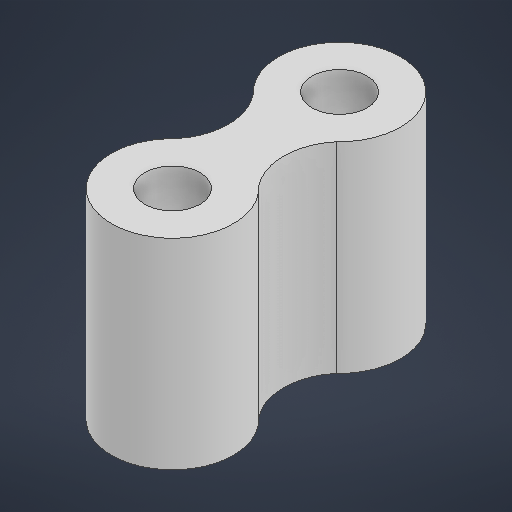
# Autodesk Inventor part: extBoardSpacer
Saved by Autodesk Inventor 2026 (Build 300175000, 175)
## iProperties
Created: 2025-05-16
Part Number: extBoardSpacer
Material: Generic
Document SubType Name: Modeling
Designer: Elizabeth
Density: 1 g/cm^3
Appearance: Default
Author: Elizabeth
Autodesk Inventor part; units mm, degrees
ref_plane "YZ Plane" through (0, 0, 0) normal (1, 0, 0) x (0, 1, 0)
ref_plane "XZ Plane" through (0, 0, 0) normal (0, 1, 0) x (-1, 0, 0)
ref_plane "XY Plane" through (0, 0, 0) normal (0, 0, 1) x (1, 0, 0)
sketch "Sketch1" plane through (0, 0, 0) normal (0, 1, 0) x (-1, 0, 0)
  circle A0 centre (0, 0) radius 1.65
  circle A1 centre (0, -10) radius 1.65
  arc A2 (-2.4786, -7.3207) -> (2.4786, -7.3207) centre (0, -10) ccw
  arc A3 (2.4786, -2.6793) -> (-2.4786, -2.6793) centre (0, 0) ccw
  arc A4 (2.8251, -2.3111) -> (2.4786, -7.3207) centre (5.3139, -5) ccw
  arc A5 (-2.4786, -7.3207) -> (-2.8251, -2.3111) centre (-5.3139, -5) ccw
  point P0 (-2.8251, -2.3111)
  dimension "d0" = 3.3
  dimension "d2" = 3.3
  dimension "d3" = 2
  dimension "d4" = 2
  constraints: 11 point on circle, 6 centre point, 1 coincident
  measures "d0" diameter of A0
  measures "d2" diameter of A1
  measures "d3" radial gap between concentric circles of A1 A2
  measures "d4" radial gap between concentric circles of A0 A3
extrude "Extrusion1" add sketch "Sketch1" along normal blind 12 contours A5 A3 A4 A2
body "Solid1"
